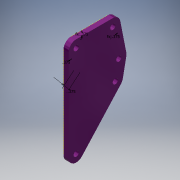
# Autodesk Inventor part: outside carriage plate
Saved by Autodesk Inventor 2017 SP1 (Build 210196100, 196)
## iProperties
Created: 2018-01-19
Part Number: outside carriage plate
Material: Aluminum 6061
Document SubType Name: Modeling
Designer: Ben
Density: 2.7 g/cm^3
Appearance: Smooth - Purple
Mass: 147.998 g
Surface Area: 209.147 cm^2
Volume: 54.8139 cm^3
Author: Ben
Autodesk Inventor part; units mm, degrees
ref_plane "YZ Plane" through (0, 0, 0) normal (1, 0, 0) x (0, 1, 0)
ref_plane "XZ Plane" through (0, 0, 0) normal (0, 1, 0) x (-1, 0, 0)
ref_plane "XY Plane" through (0, 0, 0) normal (0, 0, 1) x (1, 0, 0)
sketch "Sketch1" plane through (0, 0, 0) normal (1, 0, 0) x (0, 1, 0)
  line L0 (-420.7503, 12.7) -> (420.7488, 12.7) construction
  line L1 (420.7488, 12.7) -> (420.7488, -12.7) construction
  line L2 (420.7488, -12.7) -> (-420.7503, -12.7) construction
  line L3 (-420.7503, -12.7) -> (-420.7503, 12.7) construction
  line L4 (0, 0) -> (0, -26.6192) construction
  circle A0 centre (0, -26.6192) radius 3.302
  circle A1 centre (38.1, 26.6192) radius 3.302
  circle A2 centre (-76.2, 26.6192) radius 3.302
  line L5 (38.1, 26.6192) -> (-76.2, 26.6192) construction
  line L6 (0, 0) -> (0, 26.6192) construction
  circle A3 centre (0, -26.6192) radius 15.875 construction
  circle A4 centre (38.1, 26.6192) radius 15.875 construction
  circle A5 centre (-76.2, 26.6192) radius 15.875 construction
  line L7 (0, -26.6192) -> (-76.2, 26.6192) construction
  arc A6 (44.45, 21.8567) -> (33.3375, 32.9692) centre (38.1, 26.6192) ccw
  arc A7 (-71.4375, 32.9692) -> (-75.9328, 18.6862) centre (-76.2, 26.6192) ccw
  line L8 (-84.1375, 10.7442) -> (-84.1375, 26.6192) construction
  line L9 (-76.2, 26.6192) -> (-76.2, 0) construction
  line L10 (38.1, 26.6192) -> (38.1, 0) construction
  line L11 (45.486, 0) -> (-84.1375, 0) construction
  line L12 (-84.1375, 0) -> (-420.7503, 0) construction
  line L13 (0, -26.6192) -> (38.1, 26.6192) construction
  line L14 (0, -26.6192) -> (0, -52.0192) construction
  line L15 (13.9446, -26.6192) -> (-16.4809, -26.6192) construction
  circle A8 centre (38.1, -19.05) radius 3.302
  line L16 (38.1, -19.05) -> (38.1, 0) construction
  arc A9 (34.6661, -26.2063) -> (44.45, -14.2875) centre (38.1, -19.05) ccw
  line L17 (10.2704, -29.4344) -> (29.6856, -25.5772)
  circle A10 centre (-22.225, -22.225) radius 3.302 projected
  arc A11 (-29.588, -19.2602) -> (-18.7846, -29.3781) centre (-22.225, -22.225) ccw
  arc A12 (-5.9037, -31.9249) -> (5.9086, -31.9195) centre (0, -26.6192) ccw
  line L18 (-66.675, 31.3817) -> (28.575, 31.3817)
  line L19 (-71.1195, 17.2599) -> (-32.405, -9.7887)
  line L20 (0, -26.6192) -> (-22.225, -22.225) construction
  line L21 (-10.2678, -29.4438) -> (-13.8046, -28.7445)
  line L22 (38.1, -19.05) -> (0, -26.6192) construction
  line L23 (42.8625, 17.0942) -> (42.8625, -9.525)
  arc A13 (44.45, 21.8567) -> (42.8625, 17.0942) centre (50.8, 17.0942) ccw
  arc A14 (42.8625, -9.525) -> (44.45, -14.2875) centre (50.8, -9.525) ccw
  arc A15 (34.6661, -26.2063) -> (29.6856, -25.5772) centre (31.2323, -33.3626) ccw
  arc A16 (10.2704, -29.4344) -> (5.9086, -31.9195) centre (11.8171, -37.2197) ccw
  arc A17 (-5.9037, -31.9249) -> (-10.2678, -29.4438) centre (-11.8074, -37.2306) ccw
  arc A18 (-13.8046, -28.7445) -> (-18.7846, -29.3781) centre (-15.3442, -36.5313) ccw
  arc A19 (-29.588, -19.2602) -> (-32.405, -9.7887) centre (-36.951, -16.2954) ccw
  arc A20 (-71.1195, 17.2599) -> (-75.9328, 18.6862) centre (-75.6656, 10.7532) ccw
  arc A21 (-71.4375, 32.9692) -> (-66.675, 31.3817) centre (-66.675, 39.3192) ccw
  arc A22 (28.575, 31.3817) -> (33.3375, 32.9692) centre (28.575, 39.3192) ccw
  point P0 (42.8625, 20.2692)
  point P1 (31.75, 31.3817)
  point P2 (-69.85, 31.3817)
  point P3 (32.7997, -24.9586)
  point P4 (7.1563, -30.0531)
  point P5 (0, -42.4942)
  point P6 (-25.1604, -14.8502)
  point P7 (-16.9193, -28.1287)
  point P8 (-7.1531, -30.0596)
  point P9 (-73.7222, 19.0783)
  point P10 (42.8625, -12.7)
  dimension "d3" = 31.75
  dimension "d0" = 25.4
  dimension "d1" = 6.604
  dimension "d2" = 13.9192
  dimension "d4" = 38.1
  dimension "d5" = 76.2
  dimension "d6" = 7.9375
  dimension "d10" = 25.4
  dimension "d14" = 6.35
  dimension "d49" = 4.7625
  dimension "d52" = 4.7625
  dimension "d53" = 4.7625
  dimension "d54" = 4.7625
  dimension "d56" = 4.7625
  constraints: 48 end point, 41 point on circle, 21 centre point, 21 tangent, 17 equal radius, 17 point on line, 12 coincident, 7 vertical, 6 parallel, 3 horizontal, 3 perpendicular, 2 collinear, 1 midpoint, 1 vertical alignment, 4 other
  measures "d0" distance of L0.end L1.end
  measures "d1" diameter of A0
  measures "d2" distance from line of L2 L4.end
  measures "d4" horizontal distance of L5.start L4.end
  measures "d5" distance from line of A2.centre L6
  measures "d6" radius of A6
  measures "d10" distance of L13.start L14.end
  measures "d14" distance from line of L2 L16.start
  measures "d49" distance between parallel lines of L5 L18
  measures "d52" distance between parallel lines of L20 L21
  measures "d53" distance between parallel lines of L17 L22
  measures "d54" distance between parallel lines of L16 L23
  measures "d56" distance between parallel lines of L7 L19
extrude "Extrusion1" add sketch "Sketch1" along normal blind 6.35
sketch "Sketch5" plane through (0, 0, 0) normal (-1, 0, 0) x (0, 0, 1)
  circle A0 centre (-22.225, -22.225) radius 3.302 construction
  circle A1 centre (-19.05, 38.1) radius 3.302 construction
  circle A2 centre (26.6192, -76.2) radius 3.302 construction
  circle A3 centre (26.6192, 38.1) radius 3.302 construction
  circle A4 centre (-26.6192, 0) radius 3.302 construction
  arc A5 (32.9692, 33.3375) -> (21.8567, 44.45) centre (26.6192, 38.1) ccw construction
  arc A6 (-14.2875, 44.45) -> (-26.2063, 34.6661) centre (-19.05, 38.1) ccw construction
  line L0 (-29.4344, 10.2704) -> (-25.5772, 29.6856) construction
  arc A7 (-31.9195, 5.9086) -> (-31.9249, -5.9037) centre (-26.6192, 0) ccw construction
  arc A8 (-29.3781, -18.7846) -> (-19.2602, -29.588) centre (-22.225, -22.225) ccw construction
  arc A9 (18.6862, -75.9328) -> (32.9692, -71.4375) centre (26.6192, -76.2) ccw construction
  line L1 (26.6192, 38.1) -> (-26.6192, 0) construction
  circle A10 centre (26.6192, -76.2) radius 3.302 construction
  line L2 (-26.6192, 0) -> (26.6192, -76.2) construction
  circle A11 centre (26.6192, 38.1) radius 3.302 construction
  line L3 (26.6192, -76.2) -> (26.6192, 38.1) construction
  arc A12 (-15.6161, 30.9437) -> (-12.7, 33.3375) centre (-19.05, 38.1) ccw
  line L4 (26.6192, 38.1) -> (-19.05, 38.1) construction
  circle A13 centre (-26.6192, 0) radius 3.302 construction
  line L5 (-19.05, 38.1) -> (-26.6192, 0) construction
  line L6 (-15.6161, 30.9437) -> (-19.6026, 10.8779)
  line L7 (-19.6026, 10.8779) -> (11.781, 33.3375)
  line L8 (11.781, 33.3375) -> (-12.7, 33.3375)
  line L9 (-0.4595, 33.3375) -> (-0.4595, 38.1) construction
  line L10 (-17.6093, 20.9108) -> (-22.2806, 21.8388) construction
  line L11 (-3.9108, 22.1077) -> (-1.1391, 18.2348) construction
  arc A14 (-34.406, -1.5396) -> (-34.4045, 1.5467) centre (-26.6192, 0) ccw construction
  line L12 (21.8567, 28.8353) -> (-18.6837, -0.1774)
  line L13 (-19.0783, -2.4778) -> (21.8567, -61.068)
  line L14 (21.8567, -61.068) -> (21.8567, 28.8353)
  line L15 (-1.1391, 18.2348) -> (1.6325, 14.3619) construction
  line L16 (21.8567, -16.1163) -> (26.6192, -16.1163) construction
  line L17 (1.3892, -31.7729) -> (-2.5149, -34.5005) construction
  arc A15 (-19.0783, -2.4778) -> (-18.6837, -0.1774) centre (-26.6192, 0) ccw
  arc A16 (17.0942, 42.8625) -> (21.8567, 44.45) centre (17.0942, 50.8) ccw projected
  line L18 (-9.525, 42.8625) -> (17.0942, 42.8625) projected
  arc A17 (-14.2875, 44.45) -> (-9.525, 42.8625) centre (-9.525, 50.8) ccw projected
  arc A18 (-25.5772, 29.6856) -> (-26.2063, 34.6661) centre (-33.3626, 31.2323) ccw projected
  arc A19 (-31.9195, 5.9086) -> (-29.4344, 10.2704) centre (-37.2197, 11.8171) ccw projected
  arc A20 (-29.4438, -10.2678) -> (-31.9249, -5.9037) centre (-37.2306, -11.8074) ccw projected
  line L19 (-28.7445, -13.8046) -> (-29.4438, -10.2678) projected
  arc A21 (-29.3781, -18.7846) -> (-28.7445, -13.8046) centre (-36.5313, -15.3442) ccw projected
  arc A22 (-9.7887, -32.405) -> (-19.2602, -29.588) centre (-16.2954, -36.951) ccw projected
  line L20 (17.2599, -71.1195) -> (-9.7887, -32.405) projected
  arc A23 (18.6862, -75.9328) -> (17.2599, -71.1195) centre (10.7532, -75.6656) ccw projected
  arc A24 (31.3817, -66.675) -> (32.9692, -71.4375) centre (39.3192, -66.675) ccw projected
  line L21 (31.3817, 28.575) -> (31.3817, -66.675) projected
  arc A25 (32.9692, 33.3375) -> (31.3817, 28.575) centre (39.3192, 28.575) ccw projected
  arc A26 (-31.9195, 5.9086) -> (-31.9249, -5.9037) centre (-26.6192, 0) ccw projected
  point P0 (0, 0)
  dimension "d48" = 4.7625
  constraints: 34 end point, 7 point on circle, 6 midpoint, 6 perpendicular, 6 point on line, 5 equal length, 5 parallel, 3 centre point, 3 coincident, 2 concentric, 2 horizontal, 2 vertical
  measures "d48" distance between parallel lines of L4 L8
extrude "Extrusion2" cut sketch "Sketch5" against normal blind 4.7625
body "Solid1"
